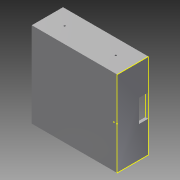
# Autodesk Inventor part: korpus
Saved by Autodesk Inventor 2014 (Build 180170000, 170)
## iProperties
Created: 2013-10-14
Part Number: korpus
Material: Stal
Document SubType Name: Modeling
Designer: Wojciech
Density: 7.85 g/cm^3
Appearance: Stal
Mass: 2020.27 g
Surface Area: 1061.32 cm^2
Volume: 257.359 cm^3
Author: Wojciech
Autodesk Inventor part; units mm, degrees
ref_plane "YZ Plane" through (0, 0, 0) normal (1, 0, 0) x (0, 1, 0)
ref_plane "XZ Plane" through (0, 0, 0) normal (0, 1, 0) x (-1, 0, 0)
ref_plane "XY Plane" through (0, 0, 0) normal (0, 0, 1) x (1, 0, 0)
sketch "Szkic1" plane through (0, 0, 0) normal (0, 1, 0) x (-1, 0, 0)
  line L0 (-75, 75) -> (75, 75)
  line L1 (75, 75) -> (75, -75)
  line L2 (75, -75) -> (-75, -75)
  line L3 (-75, -75) -> (-75, 75)
  line L4 (-75, 75) -> (75, -75) construction
  line L5 (75, 75) -> (-75, -75) construction
  point P0 (0, 0)
  dimension "d0" = 150
  dimension "d1" = 150
  constraints: 12 end point, 2 midpoint, 2 parallel, 1 horizontal, 1 perpendicular
  measures "d0" distance of L1.end L2.end
  measures "d1" distance of L0.end L1.end
extrude "Wyciągnięcie proste1" add sketch "Szkic1" along normal blind 5
sketch "Szkic2" plane through (75, 0, 75) normal (1, 0, 0) x (0, 0, -1)
  line L0 (0, 5) -> (150, 5)
  line L1 (150, 5) -> (150, 55)
  line L2 (150, 55) -> (0, 55)
  line L3 (0, 55) -> (0, 5)
  line L4 (50, 55) -> (100, 55)
  point P0 (75, 0)
  dimension "d4" = 50
  constraints: 10 end point, 2 horizontal, 2 parallel, 1 perpendicular
  measures "d4" distance of L1.end L0.end
extrude "Wyciągnięcie proste2" add sketch "Szkic2" against normal blind 5
sketch "Szkic3" plane through (-75, 0, -75) normal (-1, 0, 0) x (0, 0, 1)
  line L0 (0, 5) -> (150, 5)
  line L1 (150, 5) -> (150, 55)
  line L2 (150, 55) -> (0, 55)
  line L3 (0, 55) -> (0, 5)
  point P0 (75, 0)
  dimension "d7" = 50
  constraints: 8 end point, 2 parallel, 1 horizontal, 1 perpendicular
  measures "d7" distance of L1.end L0.end
extrude "Wyciągnięcie proste3" add sketch "Szkic3" against normal blind 5
sketch "Szkic4" plane through (-75, 0, 75) normal (0, 0, 1) x (1, 0, 0)
  line L0 (5, 5) -> (145, 5)
  line L1 (145, 5) -> (145, 55)
  line L2 (145, 55) -> (5, 55)
  line L3 (5, 55) -> (5, 5)
  point P0 (75, 0)
  constraints: 8 end point, 2 parallel, 1 horizontal, 1 perpendicular
extrude "Wyciągnięcie proste4" add sketch "Szkic4" against normal blind 5
sketch "Szkic5" plane through (75, 0, -75) normal (0, 0, -1) x (-1, 0, 0)
  line L0 (5, 5) -> (145, 5)
  line L1 (145, 5) -> (145, 55)
  line L2 (145, 55) -> (5, 55)
  line L3 (5, 55) -> (5, 5)
  point P0 (75, 0)
  constraints: 8 end point, 2 parallel, 1 horizontal, 1 perpendicular
extrude "Wyciągnięcie proste5" add sketch "Szkic5" against normal blind 5
sketch "Szkic10" plane through (-75, 0, 75) normal (0, 0, 1) x (1, 0, 0)
  circle A0 centre (30, 28) radius 1.5
  circle A1 centre (120, 28) radius 1.5
  point P0 (75, 0)
  dimension "d53" = 3
  dimension "d54" = 3
  constraints: 2 centre point
  measures "d53" diameter of A0
  measures "d54" diameter of A1
hole "Otwór5" at (45, 28, 75) at (-45, 28, 75) direction (0, 0, -1) diameter 3 depth 8 tip angle 118
sketch "Szkic11" plane through (75, 0, -75) normal (0, 0, -1) x (-1, 0, 0)
  circle A0 centre (30, 28) radius 1.5
  circle A1 centre (120, 28) radius 1.5
  point P0 (75, 0)
  dimension "d62" = 3
  dimension "d63" = 3
  constraints: 2 centre point
  measures "d62" diameter of A0
  measures "d63" diameter of A1
hole "Otwór6" at (45, 28, -75) at (-45, 28, -75) direction (0, 0, 1) diameter 3 depth 8 tip angle 118
sketch "Szkic12" plane through (70, 0, 75) normal (-1, 0, 0) x (0, 0, 1)
  line L0 (-145, 55) -> (-145, 5) projected
  line L1 (-5, 5) -> (-145, 5) projected
  line L2 (-5, 5) -> (-5, 55) projected
  line L3 (-5, 55) -> (-145, 55) projected
  point P0 (-75, 0)
sketch "Szkic13" plane through (75, 0, 75) normal (1, 0, 0) x (0, 0, -1)
  line L0 (150, 0) -> (0, 0) projected
  line L1 (150, 0) -> (150, 55) projected
  line L2 (150, 55) -> (0, 55) projected
  line L3 (0, 0) -> (0, 55) projected
  point P0 (75, 0)
sketch "Szkic14" plane through (75, 0, 75) normal (1, 0, 0) x (0, 0, -1)
  line L0 (150, 55) -> (0, 55) projected
  line L1 (55, 55) -> (95, 55)
  line L2 (95, 55) -> (95, 39)
  line L3 (95, 39) -> (55, 39)
  line L4 (55, 39) -> (55, 55)
  point P0 (75, 0)
  dimension "d73" = 40
  dimension "d74" = 16
  constraints: 8 end point, 2 parallel, 1 horizontal, 1 perpendicular, 1 point on line
  measures "d73" distance of L2.end L3.end
  measures "d74" distance of L1.end L2.end
extrude "Wyciągnięcie proste6" cut sketch "Szkic14" against normal blind 5
sketch "Szkic15" plane through (75, 0, -75) normal (0, 0, -1) x (-1, 0, 0)
  line L0 (150, 55) -> (0, 55) projected
  line L1 (55, 55) -> (95, 55)
  line L2 (95, 55) -> (95, 39)
  line L3 (95, 39) -> (55, 39)
  line L4 (55, 39) -> (55, 55)
  point P0 (75, 0)
  dimension "d77" = 40
  dimension "d78" = 16
  constraints: 8 end point, 2 parallel, 1 horizontal, 1 perpendicular, 1 point on line
  measures "d77" distance of L2.end L3.end
  measures "d78" distance of L1.end L2.end
extrude "Wyciągnięcie proste7" cut sketch "Szkic15" against normal blind 5
sketch "Szkic16" plane through (-75, 0, 75) normal (0, 0, 1) x (1, 0, 0)
  line L0 (150, 55) -> (0, 55) projected
  line L1 (55, 55) -> (95, 55)
  line L2 (95, 55) -> (95, 39)
  line L3 (95, 39) -> (55, 39)
  line L4 (55, 39) -> (55, 55)
  point P0 (75, 0)
  dimension "d81" = 40
  dimension "d82" = 16
  constraints: 8 end point, 2 parallel, 1 horizontal, 1 perpendicular, 1 point on line
  measures "d81" distance of L2.end L3.end
  measures "d82" distance of L1.end L2.end
extrude "Wyciągnięcie proste8" cut sketch "Szkic16" against normal blind 5
sketch "Szkic17" plane through (-75, 0, -75) normal (-1, 0, 0) x (0, 0, 1)
  line L0 (150, 55) -> (0, 55) projected
  line L1 (55, 55) -> (95, 55)
  line L2 (95, 55) -> (95, 39)
  line L3 (95, 39) -> (55, 39)
  line L4 (55, 39) -> (55, 55)
  point P0 (75, 0)
  dimension "d85" = 40
  dimension "d86" = 16
  constraints: 8 end point, 2 parallel, 1 horizontal, 1 perpendicular, 1 point on line
  measures "d85" distance of L2.end L3.end
  measures "d86" distance of L1.end L2.end
extrude "Wyciągnięcie proste9" cut sketch "Szkic17" against normal blind 5
